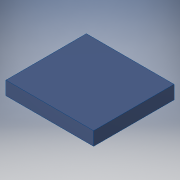
# Autodesk Inventor part: class D Amp
Saved by Autodesk Inventor 2018 (Build 220112000, 112)
## iProperties
Created: 2017-05-31
Part Number: class D Amp
Material: ABS Plastic
Document SubType Name: Modeling
Designer: Rishi
Density: 1.06 g/cm^3
Appearance: Smooth - White
Author: Rishi
Autodesk Inventor part; units mm, degrees
ref_plane "YZ Plane" through (0, 0, 0) normal (1, 0, 0) x (0, 1, 0)
ref_plane "XZ Plane" through (0, 0, 0) normal (0, 1, 0) x (-1, 0, 0)
ref_plane "XY Plane" through (0, 0, 0) normal (0, 0, 1) x (1, 0, 0)
sketch "Sketch1" plane through (0, 0, 0) normal (0, 1, 0) x (-1, 0, 0)
  line L0 (19.4, 17.8) -> (0, 17.8)
  line L1 (0, 17.8) -> (0, 0)
  line L2 (0, 0) -> (19.4, 0)
  line L3 (19.4, 0) -> (19.4, 17.8)
  dimension "d0" = 19.4
  dimension "d1" = 17.8
  constraints: 8 end point, 2 parallel, 1 horizontal, 1 perpendicular
  measures "d0" distance of L0.start L0.end
  measures "d1" distance of L2.end L0.start
extrude "Extrusion1" add sketch "Sketch1" along normal blind 3
body "Solid1"
